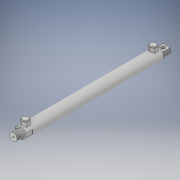
# Autodesk Inventor part: RobotArm Cylinder
Saved by Autodesk Inventor 2018 (Build 220112000, 112)
## iProperties
Created: 2018-01-15
Part Number: RobotArm Cylinder
Material: Generic
Document SubType Name: Modeling
Designer: lopez.xavier
Density: 1 g/cm^3
Appearance: Default
Author: lopez.xavier
Autodesk Inventor part; units mm, degrees
ref_plane "YZ Plane" through (0, 0, 0) normal (1, 0, 0) x (0, 1, 0)
ref_plane "XY Plane" through (0, 0, 0) normal (0, 0, 1) x (1, 0, 0)
sketch "Sketch1" plane through (0, 0, 0) normal (0, 0, 1) x (1, 0, 0)
  circle A0 centre (0, 0) radius 10.287
  dimension "d0" = 20.574
  constraints: 1 centre point, 1 coincident
  measures "d0" diameter of A0
extrude "Extrusion1" add sketch "Sketch1" along normal blind 254
ref_plane "Work Plane1" through (0, 10.287, 0) normal (0, 1, 0) x (-1, 0, 0)
sketch "Sketch2" plane through (0, 10.287, 0) normal (0, 1, 0) x (-1, 0, 0)
  line L0 (5.715, 241.8104) -> (0, 238.5109)
  line L1 (0, 238.5109) -> (-5.715, 241.8104)
  line L2 (-5.715, 241.8104) -> (-5.715, 248.4096)
  line L3 (-5.715, 248.4096) -> (0, 251.7091)
  line L4 (0, 251.7091) -> (5.715, 248.4096)
  line L5 (5.715, 248.4096) -> (5.715, 241.8104)
  line L6 (5.715, 5.5904) -> (0, 2.2909)
  line L7 (0, 2.2909) -> (-5.715, 5.5904)
  line L8 (-5.715, 5.5904) -> (-5.715, 12.1896)
  line L9 (-5.715, 12.1896) -> (0, 15.4891)
  line L10 (0, 15.4891) -> (5.715, 12.1896)
  line L11 (5.715, 12.1896) -> (5.715, 5.5904)
  line L12 (10.287, 0) -> (10.287, 254) projected
  line L13 (10.287, 254) -> (-10.287, 254) projected
  line L14 (-10.287, 0) -> (10.287, 0) projected
  point P0 (0, 0)
  point P1 (0, 245.11)
  point P2 (0, 8.89)
  dimension "d3" = 11.43
  dimension "d4" = 11.43
  dimension "d5" = 8.89
  dimension "d6" = 8.89
  dimension "d7" = 10.287
  dimension "d8" = 10.287
  constraints: 24 end point, 2 parallel, 26 other
  measures "d3" distance between parallel lines of L2 L5
  measures "d4" distance between parallel lines of L8 L11
  measures "d5" distance from line of L13 point (0, 245.11)
  measures "d6" distance from line of L14 point (0, 8.89)
  measures "d7" distance from line of L12 point (0, 245.11)
  measures "d8" distance from line of L12 point (0, 8.89)
extrude "Extrusion2" add sketch "Sketch2" along normal mid plane 12.7
sketch "Sketch3" plane through (0, 16.637, 0) normal (0, 1, 0) x (1, 0, 0)
  line L0 (0, -2.2909) -> (-5.715, -5.5904) projected
  line L1 (-5.715, -5.5904) -> (-5.715, -12.1896) projected
  line L2 (-5.715, -12.1896) -> (0, -15.4891) projected
  line L3 (0, -15.4891) -> (5.715, -12.1896) projected
  line L4 (5.715, -12.1896) -> (5.715, -5.5904) projected
  line L5 (5.715, -5.5904) -> (0, -2.2909) projected
  line L6 (0, -238.5109) -> (-5.715, -241.8104) projected
  line L7 (-5.715, -241.8104) -> (-5.715, -248.4096) projected
  line L8 (-5.715, -248.4096) -> (0, -251.7091) projected
  line L9 (0, -251.7091) -> (5.715, -248.4096) projected
  line L10 (5.715, -248.4096) -> (5.715, -241.8104) projected
  line L11 (5.715, -241.8104) -> (0, -238.5109) projected
  circle A0 centre (0, -245.1051) radius 5.08
  circle A1 centre (0, -8.8949) radius 5.08
  point P0 (0, 0)
  dimension "d11" = 10.16
  dimension "d12" = 10.16
  dimension "d13" = 5.715
  dimension "d14" = 5.715
  dimension "d15" = 6.604
  dimension "d16" = 6.604
  constraints: 2 centre point
  measures "d11" diameter of A0
  measures "d12" diameter of A1
  measures "d13" distance from line of L7 A0.centre
  measures "d14" distance from line of L1 A1.centre
  measures "d15" distance of L0.start A1.centre
  measures "d16" distance of L8.end A0.centre
extrude "Extrusion3" add sketch "Sketch3" along normal blind 2.1209 contours A0 | A1
sketch "Sketch6" plane through (0, 0, 0) normal (0, 0, -1) x (-1, 0, 0)
  circle A0 centre (0, 0) radius 10.287 projected
  circle A1 centre (0, 0) radius 7.9375
  dimension "d33" = 15.875
  constraints: 1 centre point, 1 coincident
  measures "d33" diameter of A1
extrude "Extrusion5" add sketch "Sketch6" along normal blind 0.254 contours A1
sketch "Sketch7" plane through (0, 0, -0.254) normal (0, 0, -1) x (-1, 0, 0)
  circle A0 centre (0, 0) radius 7.9375 projected
  line L0 (0, 16.637) -> (5.715, 16.637) projected
  line L1 (-6.5762, 4.445) -> (6.5762, 4.445)
  line L2 (-6.5762, -4.445) -> (6.5762, -4.445)
  arc A1 (-6.5762, 4.445) -> (-6.5762, -4.445) centre (0, 0) ccw
  arc A2 (6.5762, -4.445) -> (6.5762, 4.445) centre (0, 0) ccw
  dimension "d42" = 0
  dimension "d44" = 8.89
  dimension "d45" = 4.445
  constraints: 7 point on circle, 4 end point, 2 centre point, 2 parallel, 1 horizontal
  measures "d42" horizontal distance of L2.end L1.end
  measures "d44" distance between parallel lines of L2 L1
  measures "d45" distance from line of A0.centre L2
thread "Thread1" size "3/4-10 UNC" class "2A" standard "ANSI Unified Screw Threads" full length
extrude "Extrusion7" add sketch "Sketch7" along normal blind 15.621 contours A0 L2 L1
sketch "Sketch8" plane through (-6.5762, 4.445, -0.254) normal (0, 1, 0) x (1, 0, 0)
  circle A0 centre (6.5737, 9.271) radius 3.175
  line L0 (13.1523, 0) -> (13.1523, 15.621) projected
  line L1 (0, 15.621) -> (13.1523, 15.621) projected
  point P0 (6.5762, -0.254)
  dimension "d48" = 6.35
  dimension "d49" = 6.5786
  dimension "d50" = 6.35
  constraints: 1 centre point
  measures "d48" diameter of A0
  measures "d49" distance from line of L0 A0.centre
  measures "d50" distance from line of L1 A0.centre
extrude "Extrusion8" cut sketch "Sketch8" against normal blind 15.621
sketch "Sketch9" plane through (0, 0, 254) normal (0, 0, 1) x (1, 0, 0)
  circle A0 centre (0, 0) radius 7.9375 projected
  circle A1 centre (0, 0) radius 7.9375
  dimension "d53" = 15.875
  constraints: 1 centre point, 1 coincident
  measures "d53" diameter of A1
extrude "Extrusion9" add sketch "Sketch9" along normal blind 2.54
sketch "Sketch10" plane through (0, 0, 254) normal (0, 0, 1) x (1, 0, 0)
  circle A0 centre (0, 0) radius 7.9375 projected
  circle A1 centre (0, 0) radius 10.287 projected
  line L0 (-9.652, 3.5583) -> (-9.652, -3.5583)
  line L1 (9.652, 3.5583) -> (9.652, -3.5583)
  line L2 (-5.715, 16.637) -> (-5.715, 8.5534) projected
  arc A2 (9.652, -3.5583) -> (9.652, 3.5583) centre (0, 0) ccw
  arc A3 (-9.652, 3.5583) -> (-9.652, -3.5583) centre (0, 0) ccw
  dimension "d58" = 19.304
  dimension "d59" = 9.652
  constraints: 8 point on circle, 4 end point, 2 centre point, 2 concentric, 2 parallel, 1 vertical
  measures "d58" distance between parallel lines of L1 L0
  measures "d59" distance from line of A1.centre L0
extrude "Extrusion10" cut sketch "Sketch10" against normal blind 12.7 contours A1 L1 | A1 L0
sketch "Sketch11" plane through (0, 0, 256.54) normal (0, 0, 1) x (1, 0, 0)
  circle A0 centre (0, 0) radius 6.985
  dimension "d62" = 13.97
  constraints: 1 centre point, 1 coincident
  measures "d62" diameter of A0
extrude "Extrusion11" add sketch "Sketch11" along normal blind 10.795
thread "Thread2" size "1/4-20 UNC" class "2A" standard "ANSI Unified Screw Threads" length 25.4 offset 1.905
sketch "Sketch12" plane through (0, 0, 267.335) normal (0, 0, 1) x (1, 0, 0)
  circle A0 centre (0, 0) radius 1.5875
  dimension "d67" = 3.175
  constraints: 1 centre point, 1 coincident
  measures "d67" diameter of A0
extrude "Extrusion12" cut sketch "Sketch12" against normal blind 187.96
equation "\"d4\" = d3"
equation "\"d6\" = d5"
equation "\"d8\" = d7"
equation "\"d14\" = d13"
equation "\"d15\" = d16"
body "Solid1"
